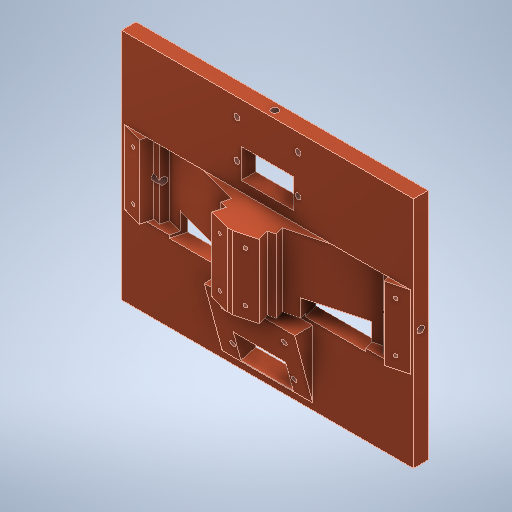
# Autodesk Inventor part: chassis_face_arriere
Saved by Autodesk Inventor 2026.2 (Build 302298010, 298A)
## iProperties
Created: 2026-03-16
Part Number: chassis_face_arriere
Material: Générique
Document SubType Name: Modeling
Designer: genon
Density: 1 g/cm^3
Appearance: Cuivre - Satiné
Author: genon
Autodesk Inventor part; units mm, degrees
ref_plane "YZ Plane" through (0, 0, 0) normal (1, 0, 0) x (0, 1, 0)
ref_plane "XZ Plane" through (0, 0, 0) normal (0, 1, 0) x (-1, 0, 0)
ref_plane "XY Plane" through (0, 0, 0) normal (0, 0, 1) x (1, 0, 0)
sketch "Esquisse1" plane through (0, 0, 0) normal (0, 0, 1) x (1, 0, 0)
  line L0 (0, 0) -> (100, 0)
  line L1 (100, 0) -> (100, 80)
  line L2 (100, 80) -> (0, 80)
  line L3 (0, 80) -> (0, 0)
  dimension "d0" = 100
  dimension "d1" = 80
  constraints: 8 end point, 2 parallel, 1 horizontal, 1 perpendicular
  measures "d0" distance of L2.end L1.end
  measures "d1" distance of L1.end L0.end
extrude "Extrusion1" add sketch "Esquisse1" against normal blind 5
sketch "Esquisse5" plane through (0, 80, 0) normal (0, 1, 0) x (1, 0, 0)
  line L0 (100, 0) -> (0, 0) projected
  line L1 (100, 5) -> (0, 5) projected
  line L2 (0, 0) -> (0, 2.5)
  line L3 (0, 0) -> (0, 5) projected
  line L4 (0, 2.5) -> (50, 2.5)
  point P0 (50, 2.5)
  dimension "d41" = 50
  constraints: 4 end point, 1 coincident, 1 midpoint, 1 perpendicular
  measures "d41" distance of L2.end L4.end
hole "Perçage3" at (50, 80, -2.5) direction (0, -1, 0) diameter 2.459 depth 8.8 tip angle 118 thread size "M3x0.5" class "6H" standard "ISO Metric profile"
sketch "Esquisse6" plane through (0, 0, 0) normal (0, -1, 0) x (1, 0, 0)
  line L0 (0, 0) -> (100, 0) projected
  line L1 (0, -5) -> (100, -5) projected
  line L2 (0, 0) -> (0, -2.5)
  line L3 (0, -2.5) -> (20, -2.5)
  line L4 (100, 0) -> (100, -5) projected
  line L5 (100, -2.5) -> (80, -2.5)
  dimension "d40" = 20
  dimension "d194" = 2.5
  dimension "d195" = 20
  constraints: 6 end point, 2 coincident, 1 horizontal, 1 midpoint, 1 perpendicular, 1 vertical
  measures "d40" distance of L2.end L3.end
  measures "d194" distance from line of L0 point (20, -2.5)
  measures "d195" distance of L5.start L5.end
hole "Perçage4" at (20, 0, -2.5) at (80, 0, -2.5) direction (0, 1, 0) diameter 2.459 depth 8.8 tip angle 118 thread size "M3x0.5" class "6H" standard "ISO Metric profile"
sketch "Esquisse7" plane through (100, 0, 0) normal (1, 0, 0) x (0, 0, -1)
  line L0 (0, 0) -> (2.5, 0)
  line L1 (0, 0) -> (5, 0) projected
  line L2 (2.5, 0) -> (2.5, 40)
  dimension "d42" = 2.5
  dimension "d43" = 40
  constraints: 4 end point, 1 coincident, 1 midpoint, 1 perpendicular
  measures "d42" distance of L0.start L0.end
  measures "d43" distance of L0.end L2.end
hole "Perçage5" at (100, 40, -2.5) direction (-1, 0, 0) diameter 2.459 depth 13 thread size "M3x0.5" class "6H" standard "ISO Metric profile"
sketch "Esquisse12" plane through (0, 0, 0) normal (-1, 0, 0) x (0, 0, 1)
  line L0 (0, 0) -> (-2.5, 0)
  line L1 (0, 0) -> (2.5, 0) construction
  line L2 (-2.5, 0) -> (-2.5, 40)
  dimension "d73" = 2.5
  dimension "d74" = 180
  dimension "d75" = 40
  constraints: 6 end point, 2 horizontal, 1 coincident, 1 collinear, 1 perpendicular
  measures "d73" distance of L0.start L0.end
  measures "d74" angle of L0 L1
  measures "d75" distance of L0.end L2.end
hole "Perçage6" at (0, 40, -2.5) direction (1, 0, 0) diameter 2.459 depth 13 thread size "M3x0.5" class "6H" standard "ISO Metric profile"
sketch "Esquisse8" plane through (0, 0, 0) normal (0, 0, 1) x (1, 0, 0)
  line L0 (100, 0) -> (0, 0) projected
  line L1 (0, 0) -> (0, 40)
  line L2 (0, 0) -> (40, 0) construction
  line L3 (0, 40) -> (100, 40)
  line L4 (0, 40) -> (100, 40) construction
  line L5 (1, 27.5) -> (49, 27.5)
  line L6 (49, 27.5) -> (49, 52.5)
  line L7 (49, 52.5) -> (1, 52.5)
  line L8 (1, 52.5) -> (1, 27.5)
  line L9 (1, 27.5) -> (49, 52.5) construction
  line L10 (49, 27.5) -> (1, 52.5) construction
  line L11 (51, 27.5) -> (99, 27.5)
  line L12 (99, 27.5) -> (99, 52.5)
  line L13 (99, 52.5) -> (51, 52.5)
  line L14 (51, 52.5) -> (51, 27.5)
  line L15 (51, 27.5) -> (99, 52.5) construction
  line L16 (99, 27.5) -> (51, 52.5) construction
  line L17 (0, 80) -> (0, 0) projected
  line L18 (100, 0) -> (100, 80) projected
  point P0 (25, 40)
  point P1 (75, 40)
  dimension "d51" = 40
  dimension "d52" = 90
  dimension "d53" = 100
  dimension "d55" = 48
  dimension "d56" = 25
  dimension "d57" = 48
  dimension "d58" = 25
  dimension "d59" = 1
  dimension "d60" = 1
  constraints: 32 end point, 5 horizontal, 4 midpoint, 4 parallel, 2 equal length, 2 perpendicular, 2 point on line, 1 vertical
  measures "d51" distance of L0.end L1.end
  measures "d52" angle of L2 L1
  measures "d53" distance of L1.end L3.end
  measures "d55" distance of L7.end L6.end
  measures "d56" distance of L6.end L5.end
  measures "d57" distance of L13.end L12.end
  measures "d58" distance of L12.end L11.end
  measures "d59" distance between parallel lines of L8 L17
  measures "d60" distance between parallel lines of L18 L12
extrude "Extrusion2" add sketch "Esquisse8" along normal blind 20 contours L12 L11 L14 L3 | L3 L14 L13 L12 | L8 L7 L6 L3 | L3 L6 L5 L8
sketch "Esquisse9" plane through (1, 52.5, 0) normal (0, 1, 0) x (1, 0, 0)
  line L0 (48, -20) -> (0, -20) projected
  line L1 (0, 0) -> (0, -20) projected
  line L2 (98, -20) -> (50, -20) projected
  line L3 (98, 0) -> (98, -20) projected
  line L4 (48, 0) -> (0, 0) projected
  line L5 (0, 0) -> (48, -12.8616)
  line L6 (48, 0) -> (48, -20) projected
  line L7 (0, 0) -> (0, -24.1525)
  line L8 (0, -24.1525) -> (48, -24.1525)
  line L9 (48, -24.1525) -> (48, -12.8616)
  line L10 (50, 0) -> (50, -20) projected
  line L11 (50, -12.8616) -> (98, 0)
  line L12 (98, 0) -> (98, -26.259)
  line L13 (98, -26.259) -> (50, -26.259)
  line L14 (50, -26.259) -> (50, -12.8616)
  point P0 (-1, 0)
  dimension "d63" = 75
  dimension "d64" = 75
  constraints: 16 end point, 3 point on line, 2 perpendicular, 1 collinear, 1 parallel, 1 vertical
  measures "d63" angle of L6 L5
  measures "d64" angle of L10 L11
extrude "Extrusion3" cut sketch "Esquisse9" against normal through all contours L0 L1 L5 L6 | L2 L10 L11 L3
sketch "Esquisse10" plane through (0, 0, 0) normal (0, 0, 1) x (1, 0, 0)
  line L0 (49, 52.5) -> (49, 27.5) projected
  line L1 (51, 27.5) -> (51, 52.5) projected
  line L2 (51, 52.5) -> (99, 52.5) projected
  line L3 (51, 52.5) -> (49, 52.5)
  line L4 (49, 27.5) -> (51, 27.5)
  point P0 (0, 0)
  constraints: 4 end point, 1 collinear, 1 parallel
extrude "Extrusion4" add sketch "Esquisse10" along normal blind 12.862
sketch "Esquisse11" plane through (1, 27.5, 0) normal (-0.258819, 0, 0.9659258) x (0.9659258, 0, 0.258819)
  line L0 (0, 25) -> (49.6933, 25) projected
  line L1 (0, 25) -> (24.8466, 25)
  line L2 (24.8466, 25) -> (9.8466, 25)
  line L3 (9.8466, 25) -> (9.8466, 0)
  line L4 (49.6933, 0) -> (0, 0) projected
  line L5 (9.8466, 0) -> (39.8466, 0)
  line L6 (39.8466, 0) -> (39.8466, 25)
  line L7 (39.8466, 25) -> (24.8466, 25)
  point P0 (-0.9659, -27.5)
  point P1 (39.8466, 0)
  point P2 (39.8466, 25)
  point P3 (9.8466, 25)
  dimension "d69" = 15
  dimension "d70" = 30
  constraints: 12 end point, 4 perpendicular, 3 point on line, 1 midpoint
  measures "d69" distance of L1.end L2.end
  measures "d70" distance of L3.end L5.end
extrude "Extrusion5" cut sketch "Esquisse11" against normal blind 7
sketch "Esquisse13" plane through (99, 27.5, 0) normal (0.258819, 0, 0.9659258) x (0.9659258, 0, -0.258819)
  line L0 (0, 25) -> (0, 0) projected
  line L1 (0, 25) -> (-24.8466, 25)
  line L2 (-49.6933, 25) -> (0, 25) projected
  line L3 (-24.8466, 25) -> (-39.8466, 25)
  line L4 (-39.8466, 25) -> (-39.8466, 0)
  line L5 (-39.8466, 0) -> (-9.8466, 0)
  line L6 (-9.8466, 0) -> (-9.8466, 25)
  line L7 (-9.8466, 25) -> (-24.8466, 25)
  point P0 (-95.6267, -27.5)
  point P1 (-9.8466, 25)
  dimension "d83" = 15
  dimension "d84" = 30
  constraints: 12 end point, 3 perpendicular, 2 point on line, 1 collinear, 1 midpoint
  measures "d83" distance of L1.end L3.end
  measures "d84" distance of L4.end L5.end
extrude "Extrusion6" cut sketch "Esquisse13" against normal blind 7
sketch "Esquisse14" plane through (1, 27.5, 0) normal (-0.258819, 0, 0.9659258) x (0.9659258, 0, 0.258819)
  line L0 (26.1244, 25) -> (68.5364, 25) projected
  line L1 (26.1244, 25) -> (2.6934, 25)
  line L2 (9.8466, 25) -> (26.1244, 25) projected
  line L3 (2.6934, 25) -> (2.6934, 22.5)
  line L4 (2.6934, 22.5) -> (47.6934, 22.5)
  line L5 (47.6934, 22.5) -> (47.6934, 2.5)
  line L6 (47.6934, 2.5) -> (2.6934, 2.5)
  line L7 (2.6934, 2.5) -> (2.6934, 22.5)
  line L8 (2.6934, 22.5) -> (2.6934, 21)
  line L9 (2.6934, 22.5) -> (4.1934, 22.5) construction
  line L10 (2.6934, 21) -> (4.1934, 21)
  line L11 (47.6934, 22.5) -> (47.6934, 21)
  line L12 (47.6934, 22.5) -> (49.1934, 22.5) construction
  line L13 (47.6934, 21) -> (46.1934, 21)
  line L14 (47.6934, 2.5) -> (47.6934, 4)
  line L15 (47.6934, 4) -> (46.1934, 4)
  line L16 (2.6934, 2.5) -> (2.6934, 4)
  line L17 (4.1934, 4) -> (2.6934, 4)
  point P0 (-0.9659, -27.5)
  point P1 (3.4434, 4)
  dimension "d87" = 23.431
  dimension "d88" = 2.5
  dimension "d89" = 45
  dimension "d90" = 20
  dimension "d91" = 1.5
  dimension "d92" = 90
  dimension "d93" = 1.5
  dimension "d94" = 1.5
  dimension "d95" = 90
  dimension "d96" = 1.5
  dimension "d97" = 1.5
  dimension "d105" = 1.5
  dimension "d106" = 1.5
  dimension "d107" = 1.5
  constraints: 32 end point, 8 perpendicular, 4 coincident, 3 collinear, 3 horizontal, 2 parallel, 2 point on line, 1 midpoint
  measures "d87" distance of L0.start L1.end
  measures "d88" distance of L1.end L3.end
  measures "d89" distance of L3.end L4.end
  measures "d90" distance of L4.end L5.end
  measures "d91" distance of L3.end L8.end
  measures "d92" angle of L8 L9
  measures "d93" distance of L8.end L10.end
  measures "d94" distance of L4.end L11.end
  measures "d95" angle of L11 L12
  measures "d96" distance of L11.end L13.end
  measures "d97" distance of L5.end L14.end
  measures "d105" distance from line of L6 point (3.443, 4)
  measures "d106" distance from line of L7 point (4.193, 4)
  measures "d107" distance of L14.end L15.end
hole "Perçage7" at (5.0505, 48.5, 1.0853) at (45.6194, 48.5, 11.9557) at (45.6194, 31.5, 11.9557) at (5.0505, 31.5, 1.0853) direction (0.258819, 0, -0.9659258) diameter 1.3211 depth 10 thread size "M1.7x0.35" class "6H" standard "ISO Metric profile"
sketch "Esquisse16" plane through (51, 27.5, 12.8616) normal (0.258819, 0, 0.9659258) x (0.9659258, 0, -0.258819)
  line L0 (0, 25) -> (9.8466, 25) projected
  line L1 (39.8466, 25) -> (49.6933, 25) projected
  line L2 (49.6933, 0) -> (39.8466, 0) projected
  line L3 (9.8466, 0) -> (0, 0) projected
  line L4 (0, 25) -> (49.6933, 25)
  line L5 (24.8466, 25) -> (1.9996, 25)
  line L6 (1.9996, 25) -> (1.9996, 22.5)
  line L7 (1.9996, 25) -> (4.4996, 25) construction
  line L8 (1.9996, 22.5) -> (46.9996, 22.5)
  line L9 (46.9996, 22.5) -> (46.9996, 2.5)
  line L10 (46.9996, 2.5) -> (1.9996, 2.5)
  line L11 (1.9996, 2.5) -> (1.9996, 22.5)
  line L12 (1.9996, 22.5) -> (46.9996, 22.5) construction
  line L13 (1.9996, 22.5) -> (1.9996, 21)
  line L14 (1.9996, 21) -> (3.4996, 21)
  line L15 (1.9996, 2.5) -> (1.9996, 4)
  line L16 (1.9996, 4) -> (3.4996, 4)
  line L17 (46.9996, 22.5) -> (46.9996, 21)
  line L18 (46.9996, 21) -> (45.4996, 21)
  line L19 (46.9996, 2.5) -> (46.9996, 4)
  line L20 (46.9996, 4) -> (45.4996, 4)
  point P0 (-45.9334, -27.5)
  dimension "d108" = 22.847
  dimension "d109" = 2.5
  dimension "d110" = 90
  dimension "d111" = 45
  dimension "d113" = 20
  dimension "d114" = 1.5
  dimension "d115" = 1.5
  dimension "d116" = 1.5
  dimension "d117" = 1.5
  constraints: 34 end point, 5 perpendicular, 5 point on line, 4 coincident, 4 horizontal, 2 equal length, 2 parallel, 1 midpoint, 1 vertical
  measures "d108" distance of L5.start L5.end
  measures "d109" distance of L5.end L6.end
  measures "d110" angle of L6 L7
  measures "d111" distance of L6.end L8.end
  measures "d113" distance of L8.end L9.end
  measures "d114" distance of L6.end L13.end
  measures "d115" distance of L13.end L14.end
  measures "d116" distance of L10.end L15.end
  measures "d117" distance of L17.end L18.end
hole "Perçage8" at (54.3804, 48.5, 11.9558) at (54.3804, 31.5, 11.9558) at (94.9493, 48.5, 1.0854) at (94.9493, 31.5, 1.0854) direction (-0.258819, 0, -0.9659258) diameter 1.3211 depth 10 thread size "M1.7x0.35" class "6H" standard "ISO Metric profile"
sketch "Esquisse17" plane through (1, 27.5, 0) normal (-0.258819, 0, 0.9659258) x (0.9659258, 0, 0.258819)
  line L0 (9.8466, 0) -> (9.8466, 25) projected
  line L1 (0, 25) -> (9.8466, 25) projected
  line L2 (9.8466, 0) -> (7.3466, 0)
  line L3 (7.3466, 0) -> (7.3466, 25)
  line L4 (7.3466, 25) -> (9.8466, 25)
  line L5 (9.8466, 25) -> (9.8466, 0)
  line L6 (39.8466, 25) -> (39.8466, 0) projected
  line L7 (39.8466, 0) -> (42.3466, 0)
  line L8 (42.3466, 0) -> (42.3466, 25)
  line L9 (42.3466, 25) -> (39.8466, 25)
  line L10 (39.8466, 25) -> (39.8466, 0)
  point P0 (-0.9659, -27.5)
  dimension "d125" = 2.5
  dimension "d126" = 2.5
  constraints: 16 end point, 4 parallel, 2 horizontal, 2 perpendicular, 2 point on line
  measures "d125" distance of L3.end L4.end
  measures "d126" distance of L9.end L8.end
extrude "Extrusion7" cut sketch "Esquisse17" against normal blind 4
sketch "Esquisse18" plane through (51, 27.5, 12.8616) normal (0.258819, 0, 0.9659258) x (0.9659258, 0, -0.258819)
  line L0 (9.8466, 0) -> (9.8466, 25) projected
  line L1 (0, 25) -> (9.8466, 25) projected
  line L2 (9.8466, 0) -> (7.3466, 0)
  line L3 (7.3466, 0) -> (7.3466, 25)
  line L4 (7.3466, 25) -> (9.8466, 25)
  line L5 (9.8466, 25) -> (9.8466, 0)
  line L6 (39.8466, 25) -> (39.8466, 0) projected
  line L7 (39.8466, 0) -> (42.3466, 0)
  line L8 (42.3466, 0) -> (42.3466, 25)
  line L9 (42.3466, 25) -> (39.8466, 25)
  line L10 (39.8466, 25) -> (39.8466, 0)
  point P0 (-45.9334, -27.5)
  point P1 (39.8466, 25)
  dimension "d129" = 2.5
  dimension "d130" = 2.5
  constraints: 16 end point, 4 parallel, 2 horizontal, 2 perpendicular, 2 point on line
  measures "d129" distance of L3.end L4.end
  measures "d130" distance of L9.end L8.end
extrude "Extrusion8" cut sketch "Esquisse18" against normal blind 4
sketch "Esquisse19" plane through (0, 0, 0) normal (0, 0, 1) x (1, 0, 0)
  line L0 (0, 0) -> (100, 0) projected
  line L1 (100, 0) -> (50, 0)
  line L2 (50, 0) -> (50, 27.5)
  line L3 (34.5, 2.25) -> (65.5, 2.25)
  line L4 (65.5, 2.25) -> (65.5, 25.25)
  line L5 (65.5, 25.25) -> (34.5, 25.25)
  line L6 (34.5, 25.25) -> (34.5, 2.25)
  line L7 (34.5, 2.25) -> (65.5, 25.25) construction
  line L8 (65.5, 2.25) -> (34.5, 25.25) construction
  point P0 (50, 13.75)
  dimension "d133" = 50
  dimension "d134" = 31
  dimension "d135" = 23
  constraints: 16 end point, 4 midpoint, 2 parallel, 1 horizontal, 1 perpendicular, 1 vertical
  measures "d133" distance of L0.end L1.end
  measures "d134" distance of L5.end L4.end
  measures "d135" distance of L4.end L3.end
extrude "Extrusion9" add sketch "Esquisse19" along normal blind 20
sketch "Esquisse20" plane through (34.5, 2.25, 0) normal (-1, 0, 0) x (0, 0, 1)
  line L0 (0, 0) -> (0, 23) projected
  line L1 (0, 0) -> (6.2226, 23.2232)
  line L2 (6.2226, 23.2232) -> (23.7957, 23.2232)
  line L3 (0, 23) -> (20, 23) projected
  line L4 (23.7957, 23.2232) -> (23.7957, -1.6817)
  line L5 (23.7957, -1.6817) -> (0, -1.6817)
  line L6 (0, -1.6817) -> (0, 0)
  point P0 (0, -2.25)
  dimension "d138" = 15
  constraints: 10 end point, 2 perpendicular, 1 parallel, 1 vertical
  measures "d138" angle of L0 L1
extrude "Extrusion10" cut sketch "Esquisse20" against normal through all contours L1 L2 L4 L5 L6
sketch "Esquisse21" plane through (34.5, 25.25, 6.1628) normal (0, -0.258819, 0.9659258) x (1, 0, 0)
  line L0 (31, -23.8114) -> (0, -23.8114) projected
  line L1 (15.5, -23.8114) -> (15.5, 0)
  line L2 (0, 0) -> (31, 0) projected
  line L3 (15.5, -11.9057) -> (28.5, -11.9057)
  line L4 (31, 0) -> (31, -23.8114) projected
  line L5 (28.5, -11.9057) -> (28.5, -2.9057)
  line L6 (28.5, -2.9057) -> (2.5, -2.9057)
  line L7 (2.5, -2.9057) -> (2.5, -20.9057)
  line L8 (2.5, -20.9057) -> (28.5, -20.9057)
  line L9 (28.5, -20.9057) -> (28.5, -11.9057)
  line L10 (2.5, -2.9057) -> (2.5, -5.4057)
  line L11 (2.5, -2.9057) -> (5, -2.9057) construction
  line L12 (2.5, -5.4057) -> (5, -5.4057)
  line L13 (2.5, -20.9057) -> (2.5, -18.4057)
  line L14 (2.5, -18.4057) -> (5, -18.4057)
  line L15 (28.5, -2.9057) -> (28.5, -5.4057)
  line L16 (28.5, -5.4057) -> (26, -5.4057)
  line L17 (28.5, -20.9057) -> (28.5, -18.4057)
  line L18 (28.5, -18.4057) -> (26, -18.4057)
  point P0 (-34.5, -25.9847)
  dimension "d141" = 13
  dimension "d142" = 9
  dimension "d143" = 26
  dimension "d144" = 18
  dimension "d145" = 2.5
  dimension "d146" = 90
  dimension "d147" = 2.5
  dimension "d148" = 2.5
  dimension "d149" = 2.5
  constraints: 32 end point, 9 perpendicular, 4 coincident, 3 horizontal, 3 midpoint, 3 point on line, 1 collinear
  measures "d141" distance of L3.start L3.end
  measures "d142" distance of L3.end L5.end
  measures "d143" distance of L5.end L6.end
  measures "d144" distance of L6.end L7.end
  measures "d145" distance of L6.end L10.end
  measures "d146" angle of L10 L11
  measures "d147" distance of L10.end L12.end
  measures "d148" distance of L7.end L13.end
  measures "d149" distance of L15.end L16.end
hole "Perçage9" at (39.5, 20.0285, 4.7637) at (60.5, 20.0285, 4.7637) at (60.5, 7.4715, 1.3991) at (39.5, 7.4715, 1.3991) direction (0, 0.258819, -0.9659258) diameter 2.013 depth 12 thread size "M2.5x0.45" class "6H" standard "ISO Metric profile"
sketch "Esquisse22" plane through (34.5, 25.25, 6.1628) normal (0, -0.258819, 0.9659258) x (1, 0, 0)
  circle A0 centre (5, -18.4057) radius 1.0065 projected
  line L0 (5, -18.4057) -> (6.5, -18.4057)
  line L1 (6.5, -18.4057) -> (6.5, -13.4057)
  line L2 (25.8927, -18.4057) -> (24.3927, -18.4057)
  line L3 (24.3927, -18.4057) -> (24.3927, -13.4057)
  line L4 (24.3927, -13.4057) -> (6.5, -13.4057)
  line L5 (24.3927, -18.4057) -> (24.3927, -23.4057)
  line L6 (24.3927, -23.4057) -> (6.5, -23.4057)
  line L7 (6.5, -23.4057) -> (6.5, -18.4057)
  point P0 (-34.5, -25.9847)
  dimension "d157" = 1.5
  dimension "d158" = 5
  dimension "d159" = 1.5
  dimension "d160" = 5
  dimension "d161" = 90
  dimension "d162" = 5
  constraints: 16 end point, 4 perpendicular, 2 horizontal, 1 point on line
  measures "d157" distance of L0.start L0.end
  measures "d158" distance of L0.end L1.end
  measures "d159" distance of L2.start L2.end
  measures "d160" distance of L2.end L3.end
  measures "d161" angle of L2 L3
  measures "d162" distance of L2.end L5.end
extrude "Extrusion11" cut sketch "Esquisse22" against normal blind 10 contours L1 L4 L3 L5 L6 L7
sketch "Esquisse23" plane through (2.8117, 27.5, -6.7615) normal (-0.258819, 0, 0.9659258) x (0.9659258, 0, 0.258819)
  line L0 (26.1244, 0) -> (9.8466, 0) projected
  line L1 (39.8466, 0) -> (39.8466, 25) projected
  line L2 (9.8466, 0) -> (39.8466, 0)
  line L3 (14.8466, -1) -> (34.8466, -1)
  line L4 (34.8466, -1) -> (34.8466, 1)
  line L5 (34.8466, 1) -> (14.8466, 1)
  line L6 (14.8466, 1) -> (14.8466, -1)
  line L7 (14.8466, -1) -> (34.8466, 1) construction
  line L8 (34.8466, -1) -> (14.8466, 1) construction
  line L9 (14.8466, 1) -> (34.8466, 1)
  line L10 (34.8466, 1) -> (34.8466, 6)
  line L11 (34.8466, 6) -> (14.8466, 6)
  line L12 (14.8466, 6) -> (14.8466, 1)
  point P0 (-0.9659, -27.5)
  point P1 (24.8466, 0)
  dimension "d165" = 20
  dimension "d166" = 2
  dimension "d167" = 5
  dimension "d170" = 20
  constraints: 22 end point, 4 parallel, 3 midpoint, 3 perpendicular, 2 horizontal
  measures "d165" distance of L5.end L4.end
  measures "d166" distance of L4.end L3.end
  measures "d167" distance of L10.end L9.end
  measures "d170" distance of L10.end L11.end
extrude "Extrusion12" cut sketch "Esquisse23" along normal through all both and the other way through all
sketch "Esquisse24" plane through (97.1883, 27.5, -6.7615) normal (0.258819, 0, 0.9659258) x (0.9659258, 0, -0.258819)
  line L0 (-9.8466, 0) -> (-26.1244, 0) projected
  line L1 (-39.8466, 25) -> (-39.8466, 0) projected
  line L2 (-9.8466, 0) -> (-39.8466, 0)
  line L3 (-34.8466, -1) -> (-14.8466, -1)
  line L4 (-14.8466, -1) -> (-14.8466, 1)
  line L5 (-14.8466, 1) -> (-34.8466, 1)
  line L6 (-34.8466, 1) -> (-34.8466, -1)
  line L7 (-34.8466, -1) -> (-14.8466, 1) construction
  line L8 (-14.8466, -1) -> (-34.8466, 1) construction
  line L9 (-34.8466, 1) -> (-14.8466, 1)
  line L10 (-14.8466, 1) -> (-14.8466, 6)
  line L11 (-14.8466, 6) -> (-34.8466, 6)
  line L12 (-34.8466, 6) -> (-34.8466, 1)
  point P0 (-95.6267, -27.5)
  point P1 (-24.8466, 0)
  point P2 (-14.8466, 1)
  dimension "d171" = 20
  dimension "d172" = 2
  dimension "d173" = 20
  dimension "d174" = 5
  constraints: 22 end point, 4 parallel, 3 midpoint, 3 perpendicular, 2 horizontal
  measures "d171" distance of L5.end L4.end
  measures "d172" distance of L4.end L3.end
  measures "d173" distance of L11.end L10.end
  measures "d174" distance of L10.end L9.end
extrude "Extrusion13" cut sketch "Esquisse24" along normal through all both and the other way through all
sketch "Esquisse25" plane through (0, 0, 0) normal (0, 0, 1) x (1, 0, 0)
  line L0 (34.5, 2.25) -> (34.5, 25.25) projected
  ellipse E0 centre (39.5, 20.0285) end of major axis (40.5065, 20.0285) minor radius 0.9722 projected
  line L1 (39.5, 20.0285) -> (39.5, 80.0996)
  ellipse E1 centre (60.5, 20.0285) end of major axis (61.5065, 20.0285) minor radius 0.9722 projected
  line L2 (60.5, 20.0285) -> (60.5, 80.0996)
  line L3 (100, 80) -> (0, 80) projected
  point P0 (0, 0)
  point P1 (39.5, 74)
  point P2 (39.5, 61)
  point P3 (60.5, 74)
  point P4 (60.5, 61)
  dimension "d177" = 13
  dimension "d178" = 13
  dimension "d179" = 21
  dimension "d180" = 6
  constraints: 4 end point, 4 point on line, 2 vertical
  measures "d177" distance of point (39.5, 61) point (39.5, 74)
  measures "d178" distance of point (60.5, 74) point (60.5, 61)
  measures "d179" distance of point (60.5, 74) point (39.5, 74)
  measures "d180" distance from line of L3 point (39.5, 74)
hole "Perçage10" at (39.5, 74, 0) at (39.5, 61, 0) at (60.5, 74, 0) at (60.5, 61, 0) direction (0, 0, -1) diameter 2.013 depth 12 thread size "M2.5x0.45" class "6H" standard "ISO Metric profile"
sketch "Esquisse26" plane through (0, 0, 0) normal (0, 0, 1) x (1, 0, 0)
  circle A0 centre (39.5, 61) radius 1.0065 projected
  line L0 (39.5, 61) -> (41, 61)
  line L1 (41, 61) -> (41, 66)
  circle A1 centre (60.5, 61) radius 1.0065 projected
  line L2 (60.5, 61) -> (59, 61)
  line L3 (59, 61) -> (59, 66)
  line L4 (59, 66) -> (41, 66)
  line L5 (59, 61) -> (59, 56)
  line L6 (59, 56) -> (41, 56)
  line L7 (41, 56) -> (41, 61)
  point P0 (0, 0)
  dimension "d188" = 1.5
  dimension "d189" = 5
  dimension "d190" = 1.5
  dimension "d191" = 5
  constraints: 16 end point, 5 perpendicular, 2 horizontal, 1 point on line
  measures "d188" distance of L0.start L0.end
  measures "d189" distance of L0.end L1.end
  measures "d190" distance of L2.start L2.end
  measures "d191" distance of L2.end L5.end
extrude "Extrusion14" cut sketch "Esquisse26" against normal blind 10 contours L1 L4 L3 L5 L6 L7
